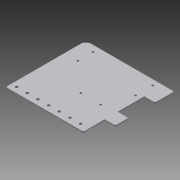
# Autodesk Inventor part: Mounting Board 3
Saved by Autodesk Inventor 2013 (Build 170138000, 138)
## iProperties
Created: 2013-01-26
Part Number: Mounting Board 3
Material: Aluminum 6061
Document SubType Name: Modeling
Designer: Moses
Mass: 325.664 g
Surface Area: 791.752 cm^2
Volume: 120.171 cm^3
Density: 2.71 g/cm^3
Author: Moses
Autodesk Inventor part; units mm, degrees
ref_plane "YZ Plane" through (0, 0, 0) normal (1, 0, 0) x (0, 1, 0)
ref_plane "XZ Plane" through (0, 0, 0) normal (0, 1, 0) x (-1, 0, 0)
ref_plane "XY Plane" through (0, 0, 0) normal (0, 0, 1) x (1, 0, 0)
sketch "Sketch1" plane through (0, 0, 0) normal (0, 1, 0) x (-1, 0, 0)
  line L0 (60.325, 101.6) -> (107.569, 101.6) construction
  circle A0 centre (60.325, 101.6) radius 2.54
  circle A1 centre (107.569, 101.6) radius 2.54
  line L1 (0, 127) -> (25.4, 127)
  line L2 (25.4, 177.8) -> (209.55, 177.8)
  line L3 (0, -12.7) -> (209.55, -12.7)
  line L4 (209.55, -12.7) -> (209.55, 177.8)
  line L5 (37.8552, 0) -> (37.8552, 40.894) construction
  circle A2 centre (37.8552, 40.894) radius 2.54
  circle A3 centre (37.8552, 0) radius 2.54
  circle A4 centre (12.7, 139.7) radius 3.302 construction
  circle A5 centre (12.7, 165.1) radius 3.302 construction
  arc A6 (23.8125, 127) -> (25.4, 128.5875) centre (23.8125, 128.5875) ccw construction
  line L6 (23.8125, 127) -> (1.5875, 127) construction
  arc A7 (0, 128.5875) -> (1.5875, 127) centre (1.5875, 128.5875) ccw construction
  line L7 (0, 128.5875) -> (0, 176.2125) construction
  arc A8 (1.5875, 177.8) -> (0, 176.2125) centre (1.5875, 176.2125) ccw construction
  line L8 (1.5875, 177.8) -> (23.8125, 177.8) construction
  arc A9 (25.4, 176.2125) -> (23.8125, 177.8) centre (23.8125, 176.2125) ccw construction
  line L9 (25.4, 176.2125) -> (25.4, 128.5875) construction
  circle A10 centre (12.7, 42.0511) radius 3.302 construction
  circle A11 centre (12.7, 86.5011) radius 3.302 construction
  line L10 (25.4, 32.5261) -> (25.4, 96.0261) projected
  line L11 (25.4, 96.0261) -> (0, 96.0261) projected
  line L12 (0, 32.5261) -> (0, 96.0261) projected
  line L13 (25.4, 32.5261) -> (0, 32.5261) projected
  circle A12 centre (69.85, 165.1) radius 3.302 projected
  circle A13 centre (196.85, 165.1) radius 3.302 projected
  circle A14 centre (146.05, 165.1) radius 3.302 projected
  circle A15 centre (120.65, 165.1) radius 3.302 projected
  line L14 (0, -12.7) -> (0, 127)
  line L15 (25.4, 177.8) -> (25.4, 127)
  circle A16 centre (44.45, 165.1) radius 3.302 projected
  circle A17 centre (95.25, 165.1) radius 3.302 projected
  circle A18 centre (171.45, 165.1) radius 3.302 projected
  line L16 (177.8, 38.481) -> (177.8, 2.413) construction
  circle A19 centre (177.8, 2.413) radius 2.54
  circle A20 centre (177.8, 38.481) radius 2.54
  line L17 (37.8552, 20.447) -> (177.8, 20.447) construction
  line L18 (37.8552, 40.894) -> (177.8, 38.481) construction
  line L19 (177.8, 2.413) -> (37.8552, 0) construction
  point P0 (0, 0)
  dimension "d8" = 47.244
  dimension "d9" = 5.08
  dimension "d21" = 40.894
  dimension "d23" = 5.08
  dimension "d24" = 12.7
  dimension "d26" = 209.55
  dimension "d29" = 34.925
  dimension "d30" = 76.2
  dimension "d31" = 190.5
  dimension "d35" = 36.068
  dimension "d37" = 31.75
  dimension "d39" = 139.9656
  constraints: 24 end point, 6 centre point, 6 coincident, 6 point on line, 4 equal radius, 3 horizontal, 2 midpoint, 2 parallel, 1 collinear, 1 vertical
  measures "d8" distance of L0.start L0.end
  measures "d9" diameter of A0
  measures "d21" distance of L5.start L5.end
  measures "d23" diameter of A2
  measures "d24" distance from line of L3 L5.start
  measures "d26" distance of L3.start L3.end
  measures "d29" distance from line of L10 A0.centre
  measures "d30" distance between parallel lines of L2 L0
  measures "d31" distance of L3.end L2.end
  measures "d35" distance of L16.end L16.start
  measures "d37" distance between parallel lines of L4 L16
  measures "d39" distance of L18.start L18.end
extrude "Extrusion1" add sketch "Sketch1" along normal blind 3.175 contours L1 L15 L2 L4 L3 L14 L13 L10 L11
fillet "Fillet1" radius 3.175 6 edges at (0, 1.5875, -12.7) (-25.4, 1.5875, 177.8) (0, 1.5875, 96.0261) (0, 1.5875, 127) (0, 1.5875, 32.5261) (-209.55, 1.5875, 177.8)
fillet "Fillet1" radius 12.7 1 edges at (-209.55, 1.5875, -12.7)
body "Solid1"
